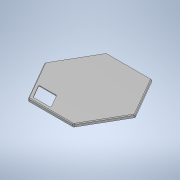
# Autodesk Inventor part: Factions_Lid
Saved by Autodesk Inventor 2021 (Build 250183000, 183)
## iProperties
Created: 2023-03-16
Part Number: Factions_Lid
Material: ABS Plastic
Document SubType Name: Modeling
Designer: Bradley
Density: 1.06 g/cm^3
Appearance: Smooth - Medium Gray
Outside: 108.400 mm
Clearance: 0.200 mm
Inside: 102.000 mm
LidDepth: 3.000 mm
FaceThickness: 1.000 mm
Author: Bradley
Autodesk Inventor part; units mm, degrees
ref_plane "YZ Plane" through (0, 0, 0) normal (1, 0, 0) x (0, 1, 0)
ref_plane "XZ Plane" through (0, 0, 0) normal (0, 1, 0) x (-1, 0, 0)
ref_plane "XY Plane" through (0, 0, 0) normal (0, 0, 1) x (1, 0, 0)
sketch "Sketch1" plane through (0, 0, 0) normal (0, 1, 0) x (-1, 0, 0)
  line L0 (-29.4449, -51) -> (-58.8897, 0)
  line L1 (-58.8897, 0) -> (-29.4449, 51)
  line L2 (-29.4449, 51) -> (29.4449, 51)
  line L3 (29.4449, 51) -> (58.8897, 0)
  line L4 (58.8897, 0) -> (29.4449, -51)
  line L5 (29.4449, -51) -> (-29.4449, -51)
  line L6 (-31.2924, -54.2) -> (-62.5848, 0)
  line L7 (-62.5848, 0) -> (-31.2924, 54.2)
  line L8 (-31.2924, 54.2) -> (31.2924, 54.2)
  line L9 (31.2924, 54.2) -> (62.5848, 0)
  line L10 (62.5848, 0) -> (31.2924, -54.2)
  line L11 (31.2924, -54.2) -> (-31.2924, -54.2)
  line L12 (-30.3109, -52.5) -> (-60.6218, 0)
  line L13 (-60.6218, 0) -> (-30.3109, 52.5)
  line L14 (-30.3109, 52.5) -> (30.3109, 52.5)
  line L15 (30.3109, 52.5) -> (60.6218, 0)
  line L16 (60.6218, 0) -> (30.3109, -52.5)
  line L17 (30.3109, -52.5) -> (-30.3109, -52.5)
  line L18 (-30.4264, -52.7) -> (-60.8527, 0)
  line L19 (-60.8527, 0) -> (-30.4264, 52.7)
  line L20 (-30.4264, 52.7) -> (30.4264, 52.7)
  line L21 (30.4264, 52.7) -> (60.8527, 0)
  line L22 (60.8527, 0) -> (30.4264, -52.7)
  line L23 (30.4264, -52.7) -> (-30.4264, -52.7)
  line L24 (0, -51) -> (0, -52.5) construction
  line L25 (0, -52.7) -> (0, -54.2) construction
  line L26 (28.8675, 50) -> (39.5485, 31.5)
  line L27 (39.5485, 31.5) -> (14.7224, 31.5)
  line L28 (14.7224, 31.5) -> (4.0415, 50)
  line L29 (4.0415, 50) -> (28.8675, 50)
  line L30 (-29.1562, 50.5) -> (29.1562, 50.5) construction
  line L31 (29.1562, 50.5) -> (58.3124, 0) construction
  line L32 (58.3124, 0) -> (29.1562, -50.5) construction
  line L33 (29.1562, -50.5) -> (-29.1562, -50.5) construction
  line L34 (-29.1562, -50.5) -> (-58.3124, 0) construction
  line L35 (-58.3124, 0) -> (-29.1562, 50.5) construction
  line L36 (40.2124, 30.35) -> (14.0007, 30.35) construction
  line L37 (14.0007, 30.35) -> (2.6558, 50) construction
  point P0 (0, 0)
  point P1 (0, 0)
  point P2 (0, 0)
  dimension "d0" = 102
  dimension "d1" = 3.2
  dimension "d2" = 0.2
  dimension "d3" = 1
  dimension "d4" = 1
  dimension "d5" = 101
  dimension "d6" = 19
  dimension "d7" = 21.5
  dimension "Outside" = 108.4
  dimension "d17" = 20.15
  dimension "d18" = 23.2
  dimension "d19" = 1.15
  dimension "d20" = 1.2
  constraints: 76 end point, 4 horizontal, 4 midpoint, 3 parallel, 2 coincident, 2 point on line, 1 collinear, 41 other
  measures "d0" distance between parallel lines of L2 L5
  measures "d1" distance between parallel lines of L5 L11
  measures "d2" distance between parallel lines of L17 L23
  measures "d3" distance between parallel lines of L2 L29
  measures "d4" distance between parallel lines of L26 L3
  measures "d5" distance between parallel lines of L30 L33
  measures "d6" distance between parallel lines of L27 L30
  measures "d7" distance between parallel lines of L28 L26
  measures "Outside" distance between parallel lines of L8 L11
  measures "d17" distance between parallel lines of L30 L36
  measures "d18" distance between parallel lines of L37 L31
  measures "d19" distance between parallel lines of L27 L36
  measures "d20" distance between parallel lines of L37 L28
extrude "Extrusion1" add sketch "Sketch1" along normal blind 1 contours L0 L1 L2 L3 L4 L5 | L6 L7 L8 L9 L10 L11 | L12 L13 L14 L15 L16 L17 | L18 L19 L20 L21 L22 L23
extrude "Extrusion2" add sketch "Sketch1" against normal blind 2.8 contours L6 L7 L8 L9 L10 L11
fillet "Fillet1" radius 2 2 edges at (-28.8675, 0.5, 50) (-14.7224, 0.5, 31.5)
fillet "Fillet1" radius 1 2 edges at (-39.5485, 0.5, 31.5) (-4.0415, 0.5, 50)
fillet "Fillet1" radius 2 6 edges at (-31.2924, -0.9, 54.2) (31.2924, -0.9, 54.2) (62.5848, -0.9, 0) (31.2924, -0.9, -54.2) (-31.2924, -0.9, -54.2) (-62.5848, -0.9, 0)
chamfer "Chamfer1" distance 1 angle 45 12 edges at (-46.9386, 1, -27.1) (-62.2754, 1, 0) (-46.9386, 1, 27.1) (-31.1377, 1, 53.9321) (0, 1, 54.2) (31.1377, 1, 53.9321) (46.9386, 1, 27.1) (62.2754, 1, 0) (46.9386, 1, -27.1) (31.1377, 1, -53.9321) (0, 1, -54.2) (-31.1377, 1, -53.9321)
equation "\"d0\" = Inside"
equation "\"d4\" = d3"
equation "\"d5\" = FlatDiameter"
equation "\"d17\" = CouncilHomeHeight"
equation "\"d18\" = CouncilHomeWidth"
equation "\"d8\" = FaceThickness"
equation "\"d10\" = LidDepth - Clearance"
equation "\"Clearance\" = 0.2"
equation "\"LidDepth\" = 3"
equation "\"FaceThickness\" = 1"
equation "\"Inside\" = 102"
equation "\"FlatDiameter\" = 101"
equation "\"CouncilHomeHeight\" = 20.15"
equation "\"CouncilHomeWidth\" = 23.2"
body "Solid1"
